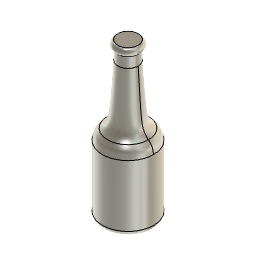
ice (Autodesk Fusion 360 design; units mm, degrees)
Autodesk Fusion 360 part; units mm, degrees
sketch "Sketch1" plane through (0, 0, 0) normal (0, 1, 0) x (1, 0, 0)
  line L0 (0, 0) -> (4, 0)
  arc A0 (5, -1) -> (4, 0) centre (4, -1) ccw
  line L1 (5, -1) -> (5, -13)
  line L2 (0, 0) -> (0, -30)
  line L3 (0, -30) -> (2, -30)
  spline S0 degree 2 poles (5, -13) (4.7977, -14.1987) (4, -15) knots 0 0 0 0.22987 0.22987 0.22987 weights 1 3 1
  arc A1 (2, -30) -> (2, -28.5) centre (1.7031, -29.25) ccw
  line L4 (2, -28.5) -> (2, -26.5)
  spline S1 degree 2 poles (4, -15) (2.6442, -16.1662) (2, -26.5) knots 0 0 0 1.18535 1.18535 1.18535 weights 1 3 1
  dimension "d1" = 4
  dimension "d2" = 12
  dimension "d3" = 30
  dimension "d9" = 2
  dimension "d11" = 2
  constraint coincident L0.start L2.start
  constraint horizontal L0
  constraint vertical L1
  constraint perpendicular L0 L2
  constraint perpendicular L2 L3
  constraint vertical L4
  measures "d1" distance of L0.start L0.end
  measures "d2" distance of A0.start L1.end
  measures "d3" distance of L0.start L2.end
  measures "d9" distance of L2.end L3.end
  measures "d11" distance of A1.end L4.end
revolve "Revolve1" add sketch "Sketch1" angle 360 about axis through (0, 0, 0) along (0, 0, 1)
